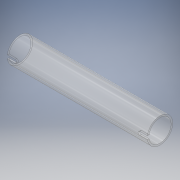
# Autodesk Inventor part: Laser_tube
Saved by Autodesk Inventor 2017 SP1 (Build 210196100, 196)
## iProperties
Created: 2016-01-13
Part Number: Laser_tube
Material: Polycarbonate, Clear
Document SubType Name: Modeling
Designer: Conor Mow-Lowry
Density: 1.2 g/cm^3
Appearance: Polycarbonate - Clear
Author: Conor Mow-Lowry
Autodesk Inventor part; units mm, degrees
ref_plane "YZ Plane" through (0, 0, 0) normal (1, 0, 0) x (0, 1, 0)
sketch "Sketch1" plane through (0, 0, 0) normal (1, 0, 0) x (0, 1, 0)
  circle A0 centre (0, 0) radius 15
  circle A1 centre (0, 0) radius 13
  dimension "d0" = 30
  dimension "d1" = 26
  constraints: 2 centre point, 2 coincident
  measures "d0" diameter of A0
  measures "d1" diameter of A1
extrude "Extrusion1" add sketch "Sketch1" along normal blind 165
sketch "Sketch2" plane through (0, 0, 0) normal (0, 1, 0) x (-1, 0, 0)
  line L0 (0, 0) -> (-165, 0) construction
  line L1 (-165, 15) -> (-165, -15) construction
  line L2 (-11, 2) -> (0, 2)
  line L3 (0, 2) -> (0, -2)
  line L4 (0, -2) -> (-11, -2)
  line L5 (-11, -2) -> (-11, 2)
  line L6 (-11, 2) -> (0, -2)
  line L7 (0, 2) -> (-11, -2)
  line L8 (0, -15) -> (0, 15) projected
  line L9 (0, 15) -> (0, -15)
  line L10 (0, -15) -> (-165, -15) projected
  point P0 (-5.5, 0)
  dimension "d4" = 4
  dimension "d5" = 11
  constraints: 16 end point, 3 midpoint, 2 parallel, 2 perpendicular, 1 collinear, 1 horizontal, 1 point on line
  measures "d4" distance of L4.end L2.start
  measures "d5" distance of L3.end L4.end
extrude "Extrusion2" cut sketch "Sketch2" against normal through all
fillet "Fillet1" radius 2 2 edges at (11, -13.8557, 2) (11, -13.8557, -2)
ref_plane "Work Plane1" through (82.5, 0, 0) normal (-1, 0, 0) x (0, 0, 1)
mirror "Mirror1" about plane through (82.5, 0, 0) normal (-1, 0, 0) of "Extrusion2", "Fillet1"
ref_plane "Work Plane2" through (0, -15, 0) normal (0, 1, 0) x (-1, 0, 0)
body "Solid1"
